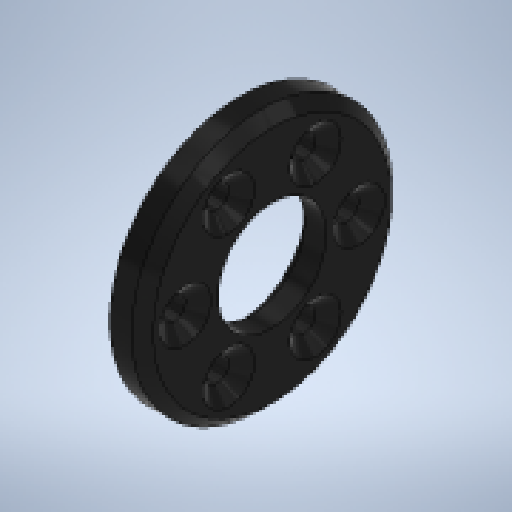
# Autodesk Inventor part: Weapon Cover
Saved by Autodesk Inventor 2023.2 (Build 272271000, 271)
## iProperties
Created: 2023-01-09
Part Number: Weapon Cover
Material: UHMW, Black
Document SubType Name: Modeling
Designer: Nathan Cai
Density: 0.94 g/cm^3
Appearance: Smooth - Black
Author: Nathan Cai
Autodesk Inventor part; units mm, degrees
ref_plane "YZ Plane" through (0, 0, 0) normal (1, 0, 0) x (0, 1, 0)
ref_plane "XZ Plane" through (0, 0, 0) normal (0, 1, 0) x (-1, 0, 0)
ref_plane "XY Plane" through (0, 0, 0) normal (0, 0, 1) x (1, 0, 0)
sketch "Sketch1" plane through (0, 0, 0) normal (0, 1, 0) x (-1, 0, 0)
  line L0 (0, 0) -> (3.175, 0)
  line L1 (3.175, 0) -> (3.175, -7.9375) construction
  line L2 (3.175, -7.9375) -> (0, -7.9375)
  line L3 (0, -7.9375) -> (0, 0)
  line L4 (3.175, 0) -> (4.7625, 0)
  line L5 (4.7625, 0) -> (4.7625, -9.525)
  line L6 (4.7625, -9.525) -> (3.175, -9.525)
  line L7 (3.175, -9.525) -> (3.175, 0)
  line L8 (0, 0) -> (4.7625, 0)
  line L9 (4.7625, 0) -> (4.7625, -19.05)
  line L10 (4.7625, -19.05) -> (0, -19.05)
  line L11 (0, -19.05) -> (0, 0)
  dimension "d0" = 3.175
  dimension "d1" = 7.9375
  dimension "d2" = 1.5875
  dimension "d3" = 9.525
  dimension "d4" = 19.05
  constraints: 24 end point, 6 parallel, 3 horizontal, 3 perpendicular, 1 midpoint
  measures "d0" distance of L1.end L2.end
  measures "d1" distance of L0.end L1.end
  measures "d2" distance of L5.end L6.end
  measures "d3" distance of L4.end L5.end
  measures "d4" distance between parallel lines of L0 L10
revolve "Revolution1" add sketch "Sketch1" angle 360 about axis through (0, 0, 0) along (-1, 0, 0) contours L2 L7 L6 L9 L10 L11
sketch "Sketch2" plane through (-4.7625, 0, 0) normal (-1, 0, 0) x (0, 0, 1)
  circle A0 centre (0, 0) radius 12.7 construction
  line L0 (0, 0) -> (-12.7, 0) construction
  circle A1 centre (-12.7, 0) radius 1.7526
  circle A2 centre (-6.35, -10.9985) radius 1.7526
  circle A3 centre (6.35, -10.9985) radius 1.7526
  circle A4 centre (12.7, 0) radius 1.7526
  circle A5 centre (6.35, 10.9985) radius 1.7526
  circle A6 centre (-6.35, 10.9985) radius 1.7526
  dimension "d6" = 25.4
  dimension "d7" = 3.5052
  dimension "d10" = 360
  constraints: 6 centre point, 2 coincident, 2 end point, 1 horizontal, 1 horizontal alignment, 15 other
  measures "d7" diameter of A1
extrude "Extrusion1" cut sketch "Sketch2" against normal blind 25.4
chamfer "Chamfer1" distance 2.032 angle 41 6 edges at (0, -10.9985, 4.5974) (0, 0, 10.9474) (0, 10.9985, 4.5974) (0, 10.9985, -8.1026) (0, 0, -14.4526) (0, -10.9985, -8.1026) measured on face at (0, 10.9985, -8.6026) measured on face at (0, 10.9985, 4.0974) measured on face at (0, -10.9985, -8.6026) measured on face at (0, -10.9985, 4.0974) measured on face at (0, 0, 10.4474) measured on face at (0, 0, -14.9526)
chamfer "Chamfer2" distance 1.5875 angle 45 1 edges at (0, 0, 19.05)
body "Solid1"
